# Autodesk Inventor part: m3_standoff_30mm
Saved by Autodesk Inventor 2022.2 (Build 262287000, 287)
## iProperties
Created: 2021-01-16
Part Number: m3_standoff_30mm
Material: Brass, Soft Yellow
Document SubType Name: Modeling
Designer: User
Density: 8.47 g/cm^3
Appearance: Brass - Satin
Author: User
Autodesk Inventor part; units mm, degrees
ref_plane "YZ Plane" through (0, 0, 0) normal (1, 0, 0) x (0, 1, 0)
ref_plane "XZ Plane" through (0, 0, 0) normal (0, 1, 0) x (-1, 0, 0)
ref_plane "XY Plane" through (0, 0, 0) normal (0, 0, 1) x (1, 0, 0)
sketch "Sketch1" plane through (0, 0, 0) normal (0, 1, 0) x (-1, 0, 0)
  line L0 (0, -2.6558) -> (-2.3, -1.3279)
  line L1 (-2.3, -1.3279) -> (-2.3, 1.3279)
  line L2 (-2.3, 1.3279) -> (0, 2.6558)
  line L3 (0, 2.6558) -> (2.3, 1.3279)
  line L4 (2.3, 1.3279) -> (2.3, -1.3279)
  line L5 (2.3, -1.3279) -> (0, -2.6558)
  circle A0 centre (0, 0) radius 1.5
  dimension "d0" = 4.6
  dimension "d1" = 3
  constraints: 12 end point, 2 coincident, 1 centre point, 1 vertical alignment, 13 other
  measures "d0" distance between parallel lines of L0 L3
  measures "d1" diameter of A0
extrude "Extrusion1" add sketch "Sketch1" along normal blind 30
sketch "Sketch2" plane through (0, 0, 0) normal (0, -1, 0) x (1, 0, 0)
  circle A0 centre (0, 0) radius 1.5 projected
extrude "Extrusion2" add sketch "Sketch2" along normal blind 4
body "Solid1"
